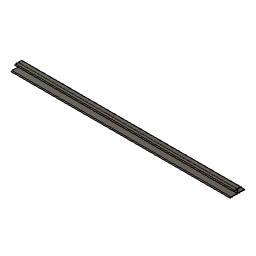
041256-1715 MH H-Shaped Retainer (Autodesk Fusion 360 design; units mm, degrees)
Autodesk Fusion 360 part; units mm, degrees
sketch "Sketch1" plane through (0, 0, 0) normal (1, 0, 0) x (0, 1, 0)
  line L0 (-0.635, 3.3734) -> (0.635, 3.3734)
  line L1 (0.635, 3.3734) -> (0.635, -3.3734)
  line L2 (0.635, -3.3734) -> (-0.635, -3.3734)
  line L3 (-0.635, -3.3734) -> (-0.635, 3.3734)
  line L4 (-0.635, 3.3734) -> (0.635, -3.3734) construction
  line L5 (0.635, 3.3734) -> (-0.635, -3.3734) construction
  line L6 (-15.367, -3.3734) -> (15.367, -3.3734)
  line L7 (15.367, -3.3734) -> (15.367, -4.6434)
  line L8 (15.367, -4.6434) -> (-15.367, -4.6434)
  line L9 (-15.367, -4.6434) -> (-15.367, -3.3734)
  line L10 (-7.9375, 4.6434) -> (7.9375, 4.6434)
  line L11 (7.9375, 4.6434) -> (7.9375, 3.3734)
  line L12 (7.9375, 3.3734) -> (-7.9375, 3.3734)
  line L13 (-7.9375, 3.3734) -> (-7.9375, 4.6434)
  point P0 (0, 3.3734)
  point P1 (0, 3.3734)
  point P2 (0, -3.3734)
  point P3 (0, -3.3734)
  dimension "d5" = 1.27
  dimension "d6" = 15.875
  dimension "d7" = 30.734
  dimension "d8" = 6.7469
  constraint horizontal L0
  constraint perpendicular L0 L1
  constraint parallel L0 L2
  constraint parallel L1 L3
  constraint coincident L4 origin
  constraint coincident L5 origin
  constraint horizontal L6
  constraint vertical L7
  constraint horizontal L8
  constraint vertical L9
  constraint horizontal L10
  constraint vertical L11
  constraint horizontal L12
  constraint vertical L13
  constraint midpoint L12 P1
  constraint midpoint L0 P1
  constraint midpoint L2 P3
  constraint midpoint L6 P3
  constraint coincident P1 P0
  constraint coincident P3 P2
  constraint equal L2 L11
  constraint equal L7 L11
  measures "d5" distance of L10.start L12.end
  measures "d6" distance of L10.start L10.end
  measures "d7" distance of L7.end L8.end
  measures "d8" distance of L0.start L2.end
extrude "Extrude1" add sketch "Sketch1" along normal mid plane 449.2625
fillet "Fillet1" radius 1.905 4 edges at (0, -15.367, -3.3734) (0, 15.367, -3.3734) (0, 7.9375, 4.6434) (0, -7.9375, 4.6434)
equation "Thickness = 0.05 in"
equation "SlotWidth = ( 17 / 64 ) * 1 in"
equation "WideSide = 1.21 in"
equation "NarrowSide = ( 5 / 8 ) * 1 in"
equation "d5 = Thickness"
equation "d6 = NarrowSide"
equation "d7 = WideSide"
equation "d8 = SlotWidth"
equation "d9 = Length"
equation "Length = 17 11/16\""
